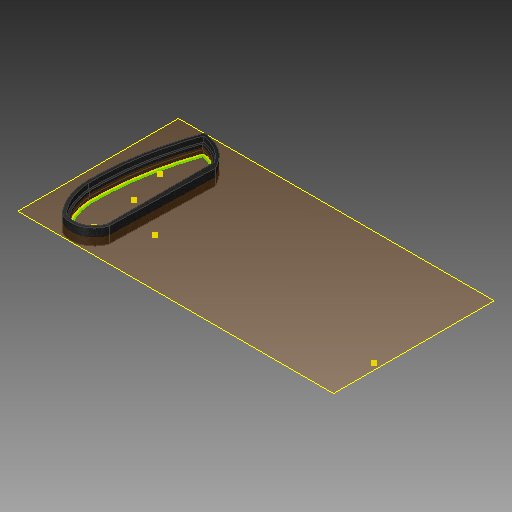
# Autodesk Inventor part: track
Saved by Autodesk Inventor 2017 (Build 210142000, 142)
## iProperties
Created: 2020-01-18
Part Number: track
Material: PBT Plastic
Document SubType Name: Modeling
Designer: Admin
Density: 1.31 g/cm^3
Appearance: Black Cast
Mass: 23.9961 g
Surface Area: 128.653 cm^2
Volume: 18.3177 cm^3
Author: Admin
Autodesk Inventor part; units mm, degrees
ref_plane "YZ Plane" through (0, 0, 0) normal (1, 0, 0) x (0, 1, 0)
ref_plane "XY Plane" through (0, 0, 0) normal (0, 0, 1) x (1, 0, 0)
sketch "Sketch1" plane through (0, 0, 0) normal (0, 1, 0) x (-1, 0, 0)
  arc A0 (24.5855, 23.6396) -> (8.8578, 61.8356) centre (-39.8212, 19.4554) ccw
  arc A1 (8.8578, 61.8356) -> (-24.5592, 49.0787) centre (-2.8694, 42.4084) ccw
  arc A2 (-27.4284, -51.6159) -> (7.5457, -75.9974) centre (10.0017, -35.1993) ccw
  arc A3 (7.5457, -75.9974) -> (24.5855, 23.6396) centre (-254.8198, 20.1477) ccw
  arc A4 (21.8724, 23.5336) -> (7.0955, 59.7239) centre (-39.8212, 19.4554) ccw
  arc A5 (7.0955, 59.7239) -> (-21.8846, 48.5356) centre (-2.8694, 42.4084) ccw
  arc A6 (-21.8846, -56.1581) -> (5.7032, -73.1142) centre (10.0017, -35.1993) ccw
  arc A7 (5.7032, -73.1142) -> (21.8724, 23.5336) centre (-254.8198, 20.1477) ccw
  line L0 (-21.8846, 48.5356) -> (-21.8846, -56.1581)
  line L1 (-24.5592, 49.0787) -> (-27.4313, -51.6092)
  arc A8 (24.5855, 23.6396) -> (8.8578, 61.8356) centre (-39.8212, 19.4554) ccw
  arc A9 (8.8578, 61.8356) -> (-24.5592, 49.0787) centre (-2.8694, 42.4084) ccw
  arc A10 (-27.4313, -51.6092) -> (7.5457, -75.9974) centre (10.0017, -35.1993) ccw
  arc A11 (7.5457, -75.9974) -> (24.5855, 23.6396) centre (-254.8198, 20.1477) ccw
  line L2 (-24.5592, 49.0787) -> (-27.4313, -51.6092)
  point P0 (0, 0)
  constraints: 27 point on circle, 12 centre point, 6 end point, 5 concentric, 1 vertical, 2 other
extrude "Extrusion1" add sketch "Sketch1" along normal blind 15.24
sketch "Sketch2" plane through (0, 0, 0) normal (0, 1, 0) x (-1, 0, 0)
  arc A0 (21.8724, 23.5336) -> (7.0955, 59.7239) centre (-39.8212, 19.4554) ccw projected
  arc A1 (5.7032, -73.1142) -> (21.8724, 23.5336) centre (-254.8198, 20.1477) ccw projected
  arc A2 (-21.8846, -56.1581) -> (5.7032, -73.1142) centre (10.0017, -35.1993) ccw projected
  line L0 (-21.8846, -56.1581) -> (-21.8846, 48.5356) projected
  arc A3 (7.0955, 59.7239) -> (-21.8846, 48.5356) centre (-2.8694, 42.4084) ccw projected
  arc A4 (20.2233, 23.4688) -> (6.03, 58.4313) centre (-39.8212, 19.4554) ccw
  arc A5 (6.03, 58.4313) -> (-20.235, 48.2707) centre (-2.8694, 42.4084) ccw
  line L1 (-20.235, 48.2707) -> (-20.235, -55.6586)
  arc A6 (-20.235, -55.6586) -> (4.5953, -71.3048) centre (10.0017, -35.1993) ccw
  arc A7 (4.5953, -71.3048) -> (20.2233, 23.4688) centre (-254.8198, 20.1477) ccw
  arc A8 (21.96, 23.537) -> (7.1522, 59.7924) centre (-39.8212, 19.4554) ccw
  arc A9 (7.1522, 59.7924) -> (-21.9723, 48.5494) centre (-2.8694, 42.4084) ccw
  line L2 (-21.9723, 48.5494) -> (-21.9723, -56.1844)
  arc A10 (-21.9723, -56.1844) -> (5.7624, -73.209) centre (10.0017, -35.1993) ccw
  arc A11 (5.7624, -73.209) -> (21.96, 23.537) centre (-254.8198, 20.1477) ccw
  point P0 (0, 0)
  constraints: 16 point on circle, 8 centre point, 4 end point, 8 other
ref_plane "Work Plane2" through (0, 7.62, 0) normal (0, 1, 0) x (-1, 0, 0)
sketch "Sketch3" plane through (0, 7.62, 0) normal (0, 1, 0) x (-1, 0, 0)
  arc A0 (21.8724, 23.5336) -> (7.0955, 59.7239) centre (-39.8212, 19.4554) ccw projected
  arc A1 (5.7032, -73.1142) -> (21.8724, 23.5336) centre (-254.8198, 20.1477) ccw projected
  arc A2 (-21.8846, -56.1581) -> (5.7032, -73.1142) centre (10.0017, -35.1993) ccw projected
  arc A3 (5.7032, -73.1142) -> (21.8724, 23.5336) centre (-254.8198, 20.1477) ccw projected
  arc A4 (-21.8846, -56.1581) -> (5.7032, -73.1142) centre (10.0017, -35.1993) ccw projected
  line L0 (-21.8846, -56.1581) -> (-21.8846, 48.5356) projected
  arc A5 (7.0955, 59.7239) -> (-21.8846, 48.5356) centre (-2.8694, 42.4084) ccw projected
  arc A6 (21.8724, 23.5336) -> (7.0955, 59.7239) centre (-39.8212, 19.4554) ccw projected
  arc A7 (8.8578, 61.8356) -> (-24.5592, 49.0787) centre (-2.8694, 42.4084) ccw projected
  line L1 (-24.5592, 49.0787) -> (-27.4313, -51.6092) projected
  arc A8 (-27.4313, -51.6092) -> (7.5457, -75.9974) centre (10.0017, -35.1993) ccw projected
  arc A9 (7.5457, -75.9974) -> (24.5855, 23.6396) centre (-254.8198, 20.1477) ccw projected
  arc A10 (24.5855, 23.6396) -> (8.8578, 61.8356) centre (-39.8212, 19.4554) ccw projected
  arc A11 (20.0927, 23.4636) -> (5.7444, 58.5644) centre (-39.8212, 19.4554) ccw
  arc A12 (4.508, -71.1594) -> (20.0927, 23.4636) centre (-254.8198, 20.1477) ccw
  arc A13 (-20.3969, -55.1802) -> (4.508, -71.1594) centre (10.0017, -35.1993) ccw
  line L2 (-20.0973, 48.248) -> (-20.0973, -55.6163)
  arc A14 (-20.0973, -55.6163) -> (4.5033, -71.1517) centre (10.0017, -35.1993) ccw
  arc A15 (4.5033, -71.1517) -> (20.0858, 23.4633) centre (-254.8198, 20.1477) ccw
  arc A16 (20.0858, 23.4633) -> (5.9414, 58.323) centre (-39.8212, 19.4554) ccw
  arc A17 (5.9414, 58.323) -> (-20.0973, 48.248) centre (-2.8694, 42.4084) ccw
  arc A18 (21.9213, 23.5355) -> (7.1272, 59.7622) centre (-39.8212, 19.4554) ccw
  arc A19 (5.7363, -73.1672) -> (21.9213, 23.5355) centre (-254.8198, 20.1477) ccw
  arc A20 (-21.9336, -56.1728) -> (5.7363, -73.1672) centre (10.0017, -35.1993) ccw
  line L3 (-21.9336, -56.1728) -> (-21.9336, 48.5433)
  arc A21 (7.1272, 59.7622) -> (-21.9336, 48.5433) centre (-2.8694, 42.4084) ccw
  point P0 (0, 0)
  constraints: 22 point on circle, 11 centre point, 4 end point, 10 other
extrude "Extrusion2" add sketch "Sketch3" along normal mid plane 5.08 contours A1 A2 L0 A5 A0
body "Solid1"
